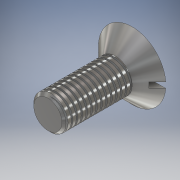
# Autodesk Inventor part: Screw
Saved by Autodesk Inventor 2018 (Build 220112000, 112)
## iProperties
Created: 2019-08-31
Part Number: Screw
Material: Generic
Document SubType Name: Modeling
Designer: HP
Density: 1 g/cm^3
Appearance: Chrome - Polished
Author: HP
Autodesk Inventor part; units mm, degrees
ref_plane "YZ Plane" through (0, 0, 0) normal (1, 0, 0) x (0, 1, 0)
ref_plane "XZ Plane" through (0, 0, 0) normal (0, 1, 0) x (-1, 0, 0)
ref_plane "XY Plane" through (0, 0, 0) normal (0, 0, 1) x (1, 0, 0)
sketch "Sketch1" plane through (0, 0, 0) normal (0, 0, 1) x (1, 0, 0)
  line L0 (0, 0) -> (0, 30)
  line L1 (0, 30) -> (12, 30)
  line L2 (12, 30) -> (6, 24)
  line L3 (12, 30) -> (23.0475, 30) construction
  line L4 (6, 24) -> (6, 0)
  line L5 (6, 0) -> (0, 0)
  dimension "d0" = 30
  dimension "d1" = 12
  dimension "d3" = 135
  constraints: 12 end point, 2 perpendicular, 2 vertical, 1 horizontal
  measures "d0" distance of L0.start L0.end
  measures "d1" distance of L0.end L1.end
  measures "d3" angle of L2 L3
revolve "Revolution1" add sketch "Sketch1" angle 360 about axis through (0, 0, 0) along (0, 1, 0)
sketch "Sketch2" plane through (0, 30, 0) normal (0, 1, 0) x (1, 0, 0)
  line L0 (-12, -1) -> (12, -1)
  line L1 (12, -1) -> (12, 1)
  line L2 (12, 1) -> (-12, 1)
  line L3 (-12, 1) -> (-12, -1)
  point P0 (0, 0)
  dimension "d5" = 2
  dimension "d6" = 1
  constraints: 8 end point, 2 parallel, 1 horizontal, 1 perpendicular
  measures "d5" distance of L2.end L0.start
  measures "d6" distance from line of point (0, 0) L2
extrude "Extrusion1" cut sketch "Sketch2" against normal blind 3
chamfer "Chamfer1" distance 1 angle 45 1 edges at (-6, 0, 0)
sketch "Sketch3" plane through (0, 0, 0) normal (0, 0, 1) x (1, 0, 0)
  line L0 (-6, 1) -> (6, 1) projected
  line L1 (-6, 0) -> (-6, -0.31)
  line L2 (-6, 0) -> (-6, 0.31)
  line L3 (-6, 0.31) -> (-5.4631, 0)
  line L4 (-6, -0.31) -> (-5.4631, 0)
  line L5 (-6, -0.31) -> (-5.3096, -0.31) construction
  point P0 (0, 0)
  dimension "d12" = 0.31
  dimension "d13" = 0.31
  dimension "d14" = 60
  dimension "d15" = 30
  constraints: 10 end point, 1 horizontal, 1 vertical
  measures "d12" distance of L1.start L1.end
  measures "d13" distance of L1.start L2.end
  measures "d14" angle of L2 L3
  measures "d15" angle of L5 L4
coil "Coil1" sketch "Sketch3" operation cut axis through (0, -10, 0) along (0, 1, 0) pitch 1.75 turns 13.714286 hand right
body "Solid1"
